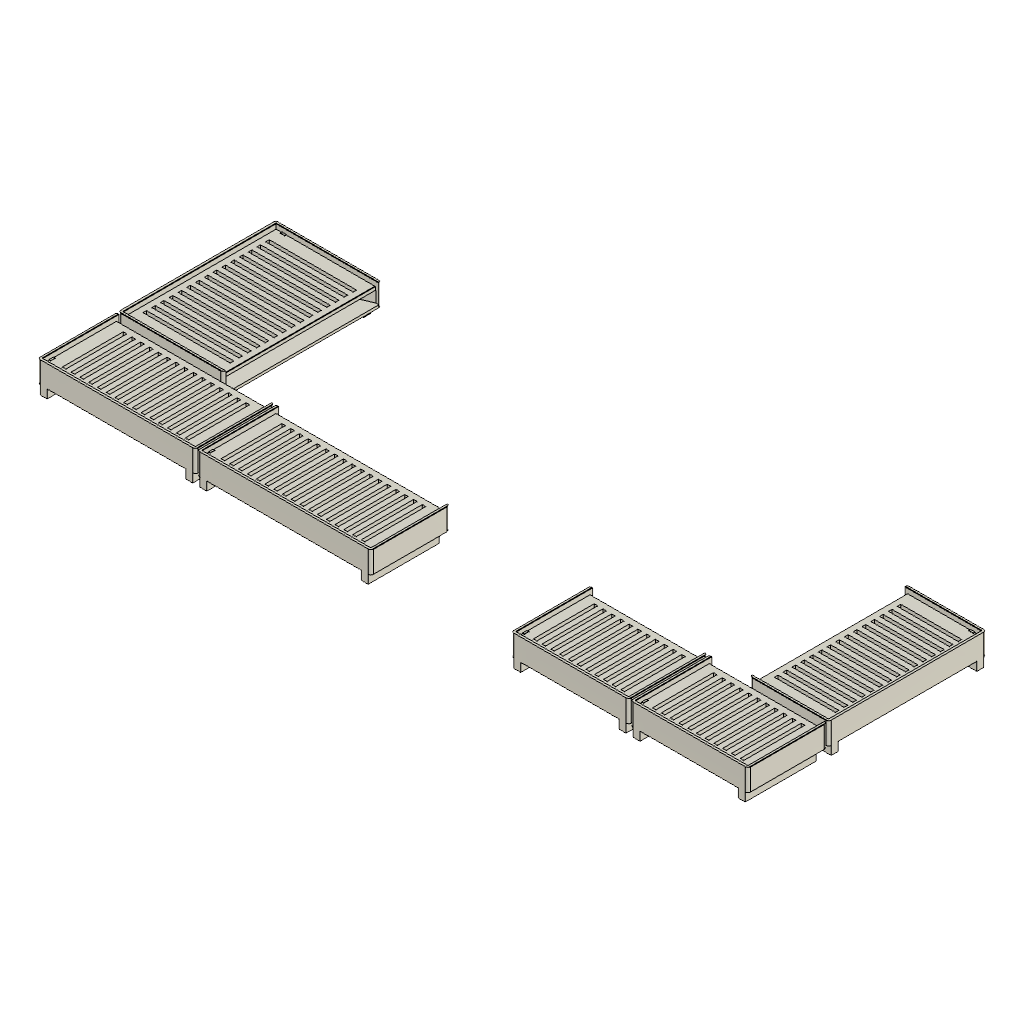
Sink_Organizer_B_R05_Flow_Rim (Autodesk Fusion 360 design; units mm, degrees)
Autodesk Fusion 360 part; units mm, degrees
(part 1 of 5)
ref_plane "工作平面1" through (0, 0, 10) normal (0, 0, 1) x (1, 0, 0) in component "R1_Integrated"
sketch "草图1" plane through (0, 0, 10) normal (0, 0, 1) x (1, 0, 0) in component "R1_Integrated"
  line L0 (590, 50) -> (724, 50)
  line L1 (724, 50) -> (724, 140)
  line L2 (724, 140) -> (590, 140)
  line L3 (590, 140) -> (590, 50)
  dimension "d47" = 590
  dimension "d48" = 50
  dimension "d49" = 134
  dimension "d50" = 90
  constraint horizontal L0
  constraint vertical L1
  constraint horizontal L2
  constraint vertical L3
  measures "d47" horizontal distance of origin L0.start
  measures "d48" vertical distance of origin L0.start
  measures "d49" horizontal distance of L0.start L0.end
  measures "d50" vertical distance of L0.end L1.end
extrude "R05 pan blank" add sketch "草图1" along normal blind 25 makes body 1 in component "R1_Integrated"
fillet "Outside corner rounds" radius 3 4 edges at (590, 140, 22.5) (724, 140, 22.5) (724, 50, 22.5) (590, 50, 22.5) on bodies 1 in component "R1_Integrated"
ref_plane "工作平面2" through (593, 0, 0) normal (1, 0, 0) x (0, 1, 0) in component "R1_Integrated"
sketch "草图2" plane through (593, 0, 0) normal (1, 0, 0) x (0, 0, -1) in component "R1_Integrated"
  line L0 (-22.1441, 53) -> (-13, 140)
  line L1 (-13, 140) -> (-36, 140)
  line L2 (-36, 140) -> (-36, 53)
  line L3 (-36, 53) -> (-22.1441, 53)
  dimension "d59" = 13
  dimension "d61" = 36
  constraint horizontal L1
  constraint vertical L2
  constraint horizontal L3
  measures "d59" horizontal distance of origin L0.end
  measures "d61" horizontal distance of origin L1.end
extrude "R05 continuous slope and open edge" cut sketch "草图2" along normal blind 128 bodies 1 in component "R1_Integrated"
ref_plane "工作平面3" through (0, 0, 10) normal (0, 0, 1) x (1, 0, 0) in component "R1_Integrated"
sketch "草图3" plane through (0, 0, 10) normal (0, 0, 1) x (1, 0, 0) in component "R1_Integrated"
  line L0 (593, 53) -> (600, 65)
  line L1 (600, 65) -> (593, 77)
  line L2 (593, 77) -> (593, 53)
  dimension "d69" = 65
  constraint vertical L2
  measures "d69" vertical distance of origin L0.end
extrude "R05 triangular flow seat 00" add sketch "草图3" along normal blind 16 bodies 1 in component "R1_Integrated"
fillet "R05 soften flow seat tip" radius 1 1 edges at (600, 65, 23.4414) on bodies 1 in component "R1_Integrated"
ref_plane "工作平面4" through (0, 0, 10) normal (0, 0, 1) x (1, 0, 0) in component "R1_Integrated"
sketch "草图4" plane through (0, 0, 10) normal (0, 0, 1) x (1, 0, 0) in component "R1_Integrated"
  line L0 (593, 113) -> (600, 125)
  line L1 (600, 125) -> (593, 137)
  line L2 (593, 137) -> (593, 113)
  dimension "d80" = 125
  constraint vertical L2
  measures "d80" vertical distance of origin L0.end
extrude "R05 triangular flow seat 01" add sketch "草图4" along normal blind 16 bodies 1 in component "R1_Integrated"
fillet "R05 soften flow seat tip (1)" radius 1 1 edges at (600, 125, 20.2883) on bodies 1 in component "R1_Integrated"
ref_plane "工作平面5" through (0, 0, 10) normal (0, 0, 1) x (1, 0, 0) in component "R1_Integrated"
sketch "草图5" plane through (0, 0, 10) normal (0, 0, 1) x (1, 0, 0) in component "R1_Integrated"
  line L0 (721, 53) -> (714, 65)
  line L1 (714, 65) -> (721, 77)
  line L2 (721, 77) -> (721, 53)
  dimension "d88" = 721
  dimension "d90" = 714
  dimension "d91" = 65
  constraint vertical L2
  measures "d88" horizontal distance of origin L0.start
  measures "d90" horizontal distance of origin L0.end
  measures "d91" vertical distance of origin L0.end
extrude "R05 triangular flow seat 10" add sketch "草图5" along normal blind 16 bodies 1 in component "R1_Integrated"
fillet "R05 soften flow seat tip (2)" radius 1 1 edges at (714, 65, 23.4414) on bodies 1 in component "R1_Integrated"
ref_plane "工作平面6" through (0, 0, 10) normal (0, 0, 1) x (1, 0, 0) in component "R1_Integrated"
sketch "草图6" plane through (0, 0, 10) normal (0, 0, 1) x (1, 0, 0) in component "R1_Integrated"
  line L0 (721, 113) -> (714, 125)
  line L1 (714, 125) -> (721, 137)
  line L2 (721, 137) -> (721, 113)
  dimension "d99" = 721
  dimension "d101" = 714
  dimension "d102" = 125
  constraint vertical L2
  measures "d99" horizontal distance of origin L0.start
  measures "d101" horizontal distance of origin L0.end
  measures "d102" vertical distance of origin L0.end
extrude "R05 triangular flow seat 11" add sketch "草图6" along normal blind 16 bodies 1 in component "R1_Integrated"
fillet "R05 soften flow seat tip (3)" radius 1 1 edges at (714, 125, 20.2883) on bodies 1 in component "R1_Integrated"
ref_plane "工作平面7" through (0, 0, 0) normal (0, 0, 1) x (1, 0, 0) in component "R1_Integrated"
sketch "草图7" plane through (0, 0, 0) normal (0, 0, 1) x (1, 0, 0) in component "R1_Integrated"
  line L0 (593, 50) -> (601, 50)
  line L1 (601, 50) -> (601, 131)
  line L2 (601, 131) -> (593, 131)
  line L3 (593, 131) -> (593, 50)
  dimension "d110" = 593
  dimension "d111" = 50
  dimension "d112" = 8
  dimension "d113" = 81
  constraint horizontal L0
  constraint vertical L1
  constraint horizontal L2
  constraint vertical L3
  measures "d110" horizontal distance of origin L0.start
  measures "d111" vertical distance of origin L0.start
  measures "d112" horizontal distance of L0.start L0.end
  measures "d113" vertical distance of L0.end L1.end
extrude "R05 low integral runner 0" add sketch "草图7" along normal blind 10 bodies 1 in component "R1_Integrated"
ref_plane "工作平面8" through (0, 0, 0) normal (0, 0, 1) x (1, 0, 0) in component "R1_Integrated"
sketch "草图8" plane through (0, 0, 0) normal (0, 0, 1) x (1, 0, 0) in component "R1_Integrated"
  line L0 (713, 50) -> (721, 50)
  line L1 (721, 50) -> (721, 131)
  line L2 (721, 131) -> (713, 131)
  line L3 (713, 131) -> (713, 50)
  dimension "d118" = 713
  dimension "d119" = 50
  dimension "d120" = 8
  dimension "d121" = 81
  constraint horizontal L0
  constraint vertical L1
  constraint horizontal L2
  constraint vertical L3
  measures "d118" horizontal distance of origin L0.start
  measures "d119" vertical distance of origin L0.start
  measures "d120" horizontal distance of L0.start L0.end
  measures "d121" vertical distance of L0.end L1.end
extrude "R05 low integral runner 1" add sketch "草图8" along normal blind 10 bodies 1 in component "R1_Integrated"
chamfer "倒角1" distance 0.4 angle 45 5 edges at (593, 96.5, 35) (721, 96.5, 35) (657, 53, 35) (590, 95, 35) (724, 95, 35) on bodies 1 in component "R1_Integrated"
ref_plane "工作平面1" through (0, 0, 26) normal (0, 0, 1) x (1, 0, 0) in component "R1_RemovableGrate"
sketch "草图1 (2)" plane through (0, 0, 26) normal (0, 0, 1) x (1, 0, 0) in component "R1_RemovableGrate"
  line L0 (593.3, 53.3) -> (720.7, 53.3)
  line L1 (720.7, 53.3) -> (720.7, 136.7)
  line L2 (720.7, 136.7) -> (593.3, 136.7)
  line L3 (593.3, 136.7) -> (593.3, 53.3)
  dimension "d129" = 127.4
  dimension "d130" = 83.4
  constraint horizontal L0
  constraint vertical L1
  constraint horizontal L2
  constraint vertical L3
  measures "d129" horizontal distance of L0.start L0.end
  measures "d130" vertical distance of L0.end L1.end
extrude "Horizontal removable deck" add sketch "草图1 (2)" along normal blind 4 separate body makes body 2 in component "R1_RemovableGrate"
ref_plane "工作平面2" through (0, 0, 26) normal (0, 0, 1) x (1, 0, 0) in component "R1_RemovableGrate"
sketch "草图2 (2)" plane through (0, 0, 26) normal (0, 0, 1) x (1, 0, 0) in component "R1_RemovableGrate"
  line L0 (605, 60.3) -> (609, 60.3)
  line L1 (609, 60.3) -> (609, 129.7)
  line L2 (609, 129.7) -> (605, 129.7)
  line L3 (605, 129.7) -> (605, 60.3)
  dimension "d135" = 605
  dimension "d137" = 4
  dimension "d138" = 69.4
  constraint horizontal L0
  constraint vertical L1
  constraint horizontal L2
  constraint vertical L3
  measures "d135" horizontal distance of origin L0.start
  measures "d137" horizontal distance of L0.start L0.end
  measures "d138" vertical distance of L0.end L1.end
extrude "Drain slot 1" cut sketch "草图2 (2)" along normal blind 4 bodies 2 in component "R1_RemovableGrate"
ref_plane "工作平面3" through (0, 0, 26) normal (0, 0, 1) x (1, 0, 0) in component "R1_RemovableGrate"
sketch "草图3 (2)" plane through (0, 0, 26) normal (0, 0, 1) x (1, 0, 0) in component "R1_RemovableGrate"
  line L0 (615, 60.3) -> (619, 60.3)
  line L1 (619, 60.3) -> (619, 129.7)
  line L2 (619, 129.7) -> (615, 129.7)
  line L3 (615, 129.7) -> (615, 60.3)
  dimension "d143" = 615
  dimension "d145" = 4
  dimension "d146" = 69.4
  constraint horizontal L0
  constraint vertical L1
  constraint horizontal L2
  constraint vertical L3
  measures "d143" horizontal distance of origin L0.start
  measures "d145" horizontal distance of L0.start L0.end
  measures "d146" vertical distance of L0.end L1.end
extrude "Drain slot 2" cut sketch "草图3 (2)" along normal blind 4 bodies 2 in component "R1_RemovableGrate"
ref_plane "工作平面4" through (0, 0, 26) normal (0, 0, 1) x (1, 0, 0) in component "R1_RemovableGrate"
sketch "草图4 (2)" plane through (0, 0, 26) normal (0, 0, 1) x (1, 0, 0) in component "R1_RemovableGrate"
  line L0 (625, 60.3) -> (629, 60.3)
  line L1 (629, 60.3) -> (629, 129.7)
  line L2 (629, 129.7) -> (625, 129.7)
  line L3 (625, 129.7) -> (625, 60.3)
  dimension "d151" = 625
  dimension "d153" = 4
  dimension "d154" = 69.4
  constraint horizontal L0
  constraint vertical L1
  constraint horizontal L2
  constraint vertical L3
  measures "d151" horizontal distance of origin L0.start
  measures "d153" horizontal distance of L0.start L0.end
  measures "d154" vertical distance of L0.end L1.end
extrude "Drain slot 3" cut sketch "草图4 (2)" along normal blind 4 bodies 2 in component "R1_RemovableGrate"
ref_plane "工作平面5" through (0, 0, 26) normal (0, 0, 1) x (1, 0, 0) in component "R1_RemovableGrate"
sketch "草图5 (2)" plane through (0, 0, 26) normal (0, 0, 1) x (1, 0, 0) in component "R1_RemovableGrate"
  line L0 (635, 60.3) -> (639, 60.3)
  line L1 (639, 60.3) -> (639, 129.7)
  line L2 (639, 129.7) -> (635, 129.7)
  line L3 (635, 129.7) -> (635, 60.3)
  dimension "d159" = 635
  dimension "d161" = 4
  dimension "d162" = 69.4
  constraint horizontal L0
  constraint vertical L1
  constraint horizontal L2
  constraint vertical L3
  measures "d159" horizontal distance of origin L0.start
  measures "d161" horizontal distance of L0.start L0.end
  measures "d162" vertical distance of L0.end L1.end
extrude "Drain slot 4" cut sketch "草图5 (2)" along normal blind 4 bodies 2 in component "R1_RemovableGrate"
ref_plane "工作平面6" through (0, 0, 26) normal (0, 0, 1) x (1, 0, 0) in component "R1_RemovableGrate"
sketch "草图6 (2)" plane through (0, 0, 26) normal (0, 0, 1) x (1, 0, 0) in component "R1_RemovableGrate"
  line L0 (645, 60.3) -> (649, 60.3)
  line L1 (649, 60.3) -> (649, 129.7)
  line L2 (649, 129.7) -> (645, 129.7)
  line L3 (645, 129.7) -> (645, 60.3)
  dimension "d167" = 645
  dimension "d169" = 4
  dimension "d170" = 69.4
  constraint horizontal L0
  constraint vertical L1
  constraint horizontal L2
  constraint vertical L3
  measures "d167" horizontal distance of origin L0.start
  measures "d169" horizontal distance of L0.start L0.end
  measures "d170" vertical distance of L0.end L1.end
extrude "Drain slot 5" cut sketch "草图6 (2)" along normal blind 4 bodies 2 in component "R1_RemovableGrate"
ref_plane "工作平面7" through (0, 0, 26) normal (0, 0, 1) x (1, 0, 0) in component "R1_RemovableGrate"
sketch "草图7 (2)" plane through (0, 0, 26) normal (0, 0, 1) x (1, 0, 0) in component "R1_RemovableGrate"
  line L0 (655, 60.3) -> (659, 60.3)
  line L1 (659, 60.3) -> (659, 129.7)
  line L2 (659, 129.7) -> (655, 129.7)
  line L3 (655, 129.7) -> (655, 60.3)
  dimension "d175" = 655
  dimension "d177" = 4
  dimension "d178" = 69.4
  constraint horizontal L0
  constraint vertical L1
  constraint horizontal L2
  constraint vertical L3
  measures "d175" horizontal distance of origin L0.start
  measures "d177" horizontal distance of L0.start L0.end
  measures "d178" vertical distance of L0.end L1.end
extrude "Drain slot 6" cut sketch "草图7 (2)" along normal blind 4 bodies 2 in component "R1_RemovableGrate"
ref_plane "工作平面8" through (0, 0, 26) normal (0, 0, 1) x (1, 0, 0) in component "R1_RemovableGrate"
sketch "草图8 (2)" plane through (0, 0, 26) normal (0, 0, 1) x (1, 0, 0) in component "R1_RemovableGrate"
  line L0 (665, 60.3) -> (669, 60.3)
  line L1 (669, 60.3) -> (669, 129.7)
  line L2 (669, 129.7) -> (665, 129.7)
  line L3 (665, 129.7) -> (665, 60.3)
  dimension "d183" = 665
  dimension "d185" = 4
  dimension "d186" = 69.4
  constraint horizontal L0
  constraint vertical L1
  constraint horizontal L2
  constraint vertical L3
  measures "d183" horizontal distance of origin L0.start
  measures "d185" horizontal distance of L0.start L0.end
  measures "d186" vertical distance of L0.end L1.end
extrude "Drain slot 7" cut sketch "草图8 (2)" along normal blind 4 bodies 2 in component "R1_RemovableGrate"
ref_plane "工作平面9" through (0, 0, 26) normal (0, 0, 1) x (1, 0, 0) in component "R1_RemovableGrate"
sketch "草图9" plane through (0, 0, 26) normal (0, 0, 1) x (1, 0, 0) in component "R1_RemovableGrate"
  line L0 (675, 60.3) -> (679, 60.3)
  line L1 (679, 60.3) -> (679, 129.7)
  line L2 (679, 129.7) -> (675, 129.7)
  line L3 (675, 129.7) -> (675, 60.3)
  dimension "d191" = 675
  dimension "d193" = 4
  dimension "d194" = 69.4
  constraint horizontal L0
  constraint vertical L1
  constraint horizontal L2
  constraint vertical L3
  measures "d191" horizontal distance of origin L0.start
  measures "d193" horizontal distance of L0.start L0.end
  measures "d194" vertical distance of L0.end L1.end
extrude "Drain slot 8" cut sketch "草图9" along normal blind 4 bodies 2 in component "R1_RemovableGrate"
ref_plane "工作平面10" through (0, 0, 26) normal (0, 0, 1) x (1, 0, 0) in component "R1_RemovableGrate"
sketch "草图10" plane through (0, 0, 26) normal (0, 0, 1) x (1, 0, 0) in component "R1_RemovableGrate"
  line L0 (685, 60.3) -> (689, 60.3)
  line L1 (689, 60.3) -> (689, 129.7)
  line L2 (689, 129.7) -> (685, 129.7)
  line L3 (685, 129.7) -> (685, 60.3)
  dimension "d199" = 685
  dimension "d201" = 4
  dimension "d202" = 69.4
  constraint horizontal L0
  constraint vertical L1
  constraint horizontal L2
  constraint vertical L3
  measures "d199" horizontal distance of origin L0.start
  measures "d201" horizontal distance of L0.start L0.end
  measures "d202" vertical distance of L0.end L1.end
extrude "Drain slot 9" cut sketch "草图10" along normal blind 4 bodies 2 in component "R1_RemovableGrate"
ref_plane "工作平面11" through (0, 0, 26) normal (0, 0, 1) x (1, 0, 0) in component "R1_RemovableGrate"
sketch "草图11" plane through (0, 0, 26) normal (0, 0, 1) x (1, 0, 0) in component "R1_RemovableGrate"
  line L0 (695, 60.3) -> (699, 60.3)
  line L1 (699, 60.3) -> (699, 129.7)
  line L2 (699, 129.7) -> (695, 129.7)
  line L3 (695, 129.7) -> (695, 60.3)
  dimension "d207" = 695
  dimension "d209" = 4
  dimension "d210" = 69.4
  constraint horizontal L0
  constraint vertical L1
  constraint horizontal L2
  constraint vertical L3
  measures "d207" horizontal distance of origin L0.start
  measures "d209" horizontal distance of L0.start L0.end
  measures "d210" vertical distance of L0.end L1.end
extrude "Drain slot 10" cut sketch "草图11" along normal blind 4 bodies 2 in component "R1_RemovableGrate"
ref_plane "工作平面12" through (0, 0, 26) normal (0, 0, 1) x (1, 0, 0) in component "R1_RemovableGrate"
sketch "草图12" plane through (0, 0, 26) normal (0, 0, 1) x (1, 0, 0) in component "R1_RemovableGrate"
  line L0 (705, 60.3) -> (709, 60.3)
  line L1 (709, 60.3) -> (709, 129.7)
  line L2 (709, 129.7) -> (705, 129.7)
  line L3 (705, 129.7) -> (705, 60.3)
  dimension "d215" = 705
  dimension "d217" = 4
  dimension "d218" = 69.4
  constraint horizontal L0
  constraint vertical L1
  constraint horizontal L2
  constraint vertical L3
  measures "d215" horizontal distance of origin L0.start
  measures "d217" horizontal distance of L0.start L0.end
  measures "d218" vertical distance of L0.end L1.end
extrude "Drain slot 11" cut sketch "草图12" along normal blind 4 bodies 2 in component "R1_RemovableGrate"
chamfer "倒角1'" distance 0.4 angle 45 4 edges at (657, 136.7, 30) (720.7, 95, 30) (657, 53.3, 30) (593.3, 95, 30) on bodies 2 in component "R1_RemovableGrate"
ref_plane "工作平面1" through (0, 0, 10) normal (0, 0, 1) x (1, 0, 0) in component "L1_Integrated"
sketch "草图1 (3)" plane through (0, 0, 10) normal (0, 0, 1) x (1, 0, 0) in component "L1_Integrated"
  line L0 (50, 50) -> (230, 50)
  line L1 (230, 50) -> (230, 140)
  line L2 (230, 140) -> (50, 140)
  line L3 (50, 140) -> (50, 50)
  dimension "d224" = 50
  dimension "d225" = 50
  dimension "d226" = 180
  dimension "d227" = 90
  constraint horizontal L0
  constraint vertical L1
  constraint horizontal L2
  constraint vertical L3
  measures "d224" horizontal distance of origin L0.start
  measures "d225" vertical distance of origin L0.start
  measures "d226" horizontal distance of L0.start L0.end
  measures "d227" vertical distance of L0.end L1.end
extrude "R05 pan blank'" add sketch "草图1 (3)" along normal blind 25 separate body makes body 3 in component "L1_Integrated"
fillet "Outside corner rounds'" radius 3 4 edges at (50, 140, 22.5) (230, 140, 22.5) (230, 50, 22.5) (50, 50, 22.5) on bodies 3 in component "L1_Integrated"
ref_plane "工作平面2" through (53, 0, 0) normal (1, 0, 0) x (0, 1, 0) in component "L1_Integrated"
sketch "草图2 (3)" plane through (53, 0, 0) normal (1, 0, 0) x (0, 0, -1) in component "L1_Integrated"
  line L0 (-22.1441, 53) -> (-13, 140)
  line L1 (-13, 140) -> (-36, 140)
  line L2 (-36, 140) -> (-36, 53)
  line L3 (-36, 53) -> (-22.1441, 53)
  dimension "d236" = 13
  dimension "d238" = 36
  constraint horizontal L1
  constraint vertical L2
  constraint horizontal L3
  measures "d236" horizontal distance of origin L0.end
  measures "d238" horizontal distance of origin L1.end
extrude "R05 continuous slope and open edge'" cut sketch "草图2 (3)" along normal blind 174 bodies 3 in component "L1_Integrated"
ref_plane "工作平面3" through (0, 0, 10) normal (0, 0, 1) x (1, 0, 0) in component "L1_Integrated"
sketch "草图3 (3)" plane through (0, 0, 10) normal (0, 0, 1) x (1, 0, 0) in component "L1_Integrated"
  line L0 (53, 53) -> (60, 65)
  line L1 (60, 65) -> (53, 77)
  line L2 (53, 77) -> (53, 53)
  dimension "d246" = 65
  constraint vertical L2
  measures "d246" vertical distance of origin L0.end
extrude "R05 triangular flow seat 00'" add sketch "草图3 (3)" along normal blind 16 bodies 3 in component "L1_Integrated"
fillet "R05 soften flow seat tip'" radius 1 1 edges at (60, 65, 23.4414) on bodies 3 in component "L1_Integrated"
ref_plane "工作平面4" through (0, 0, 10) normal (0, 0, 1) x (1, 0, 0) in component "L1_Integrated"
sketch "草图4 (3)" plane through (0, 0, 10) normal (0, 0, 1) x (1, 0, 0) in component "L1_Integrated"
  line L0 (53, 113) -> (60, 125)
  line L1 (60, 125) -> (53, 137)
  line L2 (53, 137) -> (53, 113)
  dimension "d257" = 125
  constraint vertical L2
  measures "d257" vertical distance of origin L0.end
extrude "R05 triangular flow seat 01'" add sketch "草图4 (3)" along normal blind 16 bodies 3 in component "L1_Integrated"
fillet "R05 soften flow seat tip (1)'" radius 1 1 edges at (60, 125, 20.2883) on bodies 3 in component "L1_Integrated"
ref_plane "工作平面5" through (0, 0, 10) normal (0, 0, 1) x (1, 0, 0) in component "L1_Integrated"
sketch "草图5 (3)" plane through (0, 0, 10) normal (0, 0, 1) x (1, 0, 0) in component "L1_Integrated"
  line L0 (227, 53) -> (220, 65)
  line L1 (220, 65) -> (227, 77)
  line L2 (227, 77) -> (227, 53)
  dimension "d268" = 65
  constraint vertical L2
  measures "d268" vertical distance of origin L0.end
extrude "R05 triangular flow seat 10'" add sketch "草图5 (3)" along normal blind 16 bodies 3 in component "L1_Integrated"
fillet "R05 soften flow seat tip (2)'" radius 1 1 edges at (220, 65, 23.4414) on bodies 3 in component "L1_Integrated"
ref_plane "工作平面6" through (0, 0, 10) normal (0, 0, 1) x (1, 0, 0) in component "L1_Integrated"
sketch "草图6 (3)" plane through (0, 0, 10) normal (0, 0, 1) x (1, 0, 0) in component "L1_Integrated"
  line L0 (227, 113) -> (220, 125)
  line L1 (220, 125) -> (227, 137)
  line L2 (227, 137) -> (227, 113)
  dimension "d279" = 125
  constraint vertical L2
  measures "d279" vertical distance of origin L0.end
extrude "R05 triangular flow seat 11'" add sketch "草图6 (3)" along normal blind 16 bodies 3 in component "L1_Integrated"
fillet "R05 soften flow seat tip (3)'" radius 1 1 edges at (220, 125, 20.2883) on bodies 3 in component "L1_Integrated"
ref_plane "工作平面7" through (0, 0, 0) normal (0, 0, 1) x (1, 0, 0) in component "L1_Integrated"
sketch "草图7 (3)" plane through (0, 0, 0) normal (0, 0, 1) x (1, 0, 0) in component "L1_Integrated"
  line L0 (53, 50) -> (61, 50)
  line L1 (61, 50) -> (61, 131)
  line L2 (61, 131) -> (53, 131)
  line L3 (53, 131) -> (53, 50)
  dimension "d287" = 53
  dimension "d288" = 50
  dimension "d289" = 8
  dimension "d290" = 81
  constraint horizontal L0
  constraint vertical L1
  constraint horizontal L2
  constraint vertical L3
  measures "d287" horizontal distance of origin L0.start
  measures "d288" vertical distance of origin L0.start
  measures "d289" horizontal distance of L0.start L0.end
  measures "d290" vertical distance of L0.end L1.end
extrude "R05 low integral runner 0'" add sketch "草图7 (3)" along normal blind 10 bodies 3 in component "L1_Integrated"
ref_plane "工作平面8" through (0, 0, 0) normal (0, 0, 1) x (1, 0, 0) in component "L1_Integrated"
sketch "草图8 (3)" plane through (0, 0, 0) normal (0, 0, 1) x (1, 0, 0) in component "L1_Integrated"
  line L0 (219, 50) -> (227, 50)
  line L1 (227, 50) -> (227, 131)
  line L2 (227, 131) -> (219, 131)
  line L3 (219, 131) -> (219, 50)
  dimension "d295" = 219
  dimension "d296" = 50
  dimension "d297" = 8
  dimension "d298" = 81
  constraint horizontal L0
  constraint vertical L1
  constraint horizontal L2
  constraint vertical L3
  measures "d295" horizontal distance of origin L0.start
  measures "d296" vertical distance of origin L0.start
  measures "d297" horizontal distance of L0.start L0.end
  measures "d298" vertical distance of L0.end L1.end
extrude "R05 low integral runner 1'" add sketch "草图8 (3)" along normal blind 10 bodies 3 in component "L1_Integrated"
chamfer "倒角1''" distance 0.4 angle 45 5 edges at (53, 96.5, 35) (227, 96.5, 35) (140, 53, 35) (50, 95, 35) (230, 95, 35) on bodies 3 in component "L1_Integrated"
ref_plane "工作平面1" through (0, 0, 26) normal (0, 0, 1) x (1, 0, 0) in component "L1_RemovableGrate"
sketch "草图1 (4)" plane through (0, 0, 26) normal (0, 0, 1) x (1, 0, 0) in component "L1_RemovableGrate"
  line L0 (53.3, 53.3) -> (226.7, 53.3)
  line L1 (226.7, 53.3) -> (226.7, 136.7)
  line L2 (226.7, 136.7) -> (53.3, 136.7)
  line L3 (53.3, 136.7) -> (53.3, 53.3)
  dimension "d306" = 173.4
  dimension "d307" = 83.4
  constraint horizontal L0
  constraint vertical L1
  constraint horizontal L2
  constraint vertical L3
  measures "d306" horizontal distance of L0.start L0.end
  measures "d307" vertical distance of L0.end L1.end
extrude "Horizontal removable deck'" add sketch "草图1 (4)" along normal blind 4 separate body makes body 4 in component "L1_RemovableGrate"
ref_plane "工作平面2" through (0, 0, 26) normal (0, 0, 1) x (1, 0, 0) in component "L1_RemovableGrate"
sketch "草图2 (4)" plane through (0, 0, 26) normal (0, 0, 1) x (1, 0, 0) in component "L1_RemovableGrate"
  line L0 (68, 60.3) -> (72, 60.3)
  line L1 (72, 60.3) -> (72, 129.7)
  line L2 (72, 129.7) -> (68, 129.7)
  line L3 (68, 129.7) -> (68, 60.3)
  dimension "d312" = 68
  dimension "d314" = 4
  dimension "d315" = 69.4
  constraint horizontal L0
  constraint vertical L1
  constraint horizontal L2
  constraint vertical L3
  measures "d312" horizontal distance of origin L0.start
  measures "d314" horizontal distance of L0.start L0.end
  measures "d315" vertical distance of L0.end L1.end
extrude "Drain slot 1'" cut sketch "草图2 (4)" along normal blind 4 bodies 4 in component "L1_RemovableGrate"
ref_plane "工作平面3" through (0, 0, 26) normal (0, 0, 1) x (1, 0, 0) in component "L1_RemovableGrate"
sketch "草图3 (4)" plane through (0, 0, 26) normal (0, 0, 1) x (1, 0, 0) in component "L1_RemovableGrate"
  line L0 (78, 60.3) -> (82, 60.3)
  line L1 (82, 60.3) -> (82, 129.7)
  line L2 (82, 129.7) -> (78, 129.7)
  line L3 (78, 129.7) -> (78, 60.3)
  dimension "d320" = 78
  dimension "d322" = 4
  dimension "d323" = 69.4
  constraint horizontal L0
  constraint vertical L1
  constraint horizontal L2
  constraint vertical L3
  measures "d320" horizontal distance of origin L0.start
  measures "d322" horizontal distance of L0.start L0.end
  measures "d323" vertical distance of L0.end L1.end
extrude "Drain slot 2'" cut sketch "草图3 (4)" along normal blind 4 bodies 4 in component "L1_RemovableGrate"
ref_plane "工作平面4" through (0, 0, 26) normal (0, 0, 1) x (1, 0, 0) in component "L1_RemovableGrate"
sketch "草图4 (4)" plane through (0, 0, 26) normal (0, 0, 1) x (1, 0, 0) in component "L1_RemovableGrate"
  line L0 (88, 60.3) -> (92, 60.3)
  line L1 (92, 60.3) -> (92, 129.7)
  line L2 (92, 129.7) -> (88, 129.7)
  line L3 (88, 129.7) -> (88, 60.3)
  dimension "d328" = 88
  dimension "d330" = 4
  dimension "d331" = 69.4
  constraint horizontal L0
  constraint vertical L1
  constraint horizontal L2
  constraint vertical L3
  measures "d328" horizontal distance of origin L0.start
  measures "d330" horizontal distance of L0.start L0.end
  measures "d331" vertical distance of L0.end L1.end
extrude "Drain slot 3'" cut sketch "草图4 (4)" along normal blind 4 bodies 4 in component "L1_RemovableGrate"
ref_plane "工作平面5" through (0, 0, 26) normal (0, 0, 1) x (1, 0, 0) in component "L1_RemovableGrate"
sketch "草图5 (4)" plane through (0, 0, 26) normal (0, 0, 1) x (1, 0, 0) in component "L1_RemovableGrate"
  line L0 (98, 60.3) -> (102, 60.3)
  line L1 (102, 60.3) -> (102, 129.7)
  line L2 (102, 129.7) -> (98, 129.7)
  line L3 (98, 129.7) -> (98, 60.3)
  dimension "d336" = 98
  dimension "d338" = 4
  dimension "d339" = 69.4
  constraint horizontal L0
  constraint vertical L1
  constraint horizontal L2
  constraint vertical L3
  measures "d336" horizontal distance of origin L0.start
  measures "d338" horizontal distance of L0.start L0.end
  measures "d339" vertical distance of L0.end L1.end
extrude "Drain slot 4'" cut sketch "草图5 (4)" along normal blind 4 bodies 4 in component "L1_RemovableGrate"
ref_plane "工作平面6" through (0, 0, 26) normal (0, 0, 1) x (1, 0, 0) in component "L1_RemovableGrate"
sketch "草图6 (4)" plane through (0, 0, 26) normal (0, 0, 1) x (1, 0, 0) in component "L1_RemovableGrate"
  line L0 (108, 60.3) -> (112, 60.3)
  line L1 (112, 60.3) -> (112, 129.7)
  line L2 (112, 129.7) -> (108, 129.7)
  line L3 (108, 129.7) -> (108, 60.3)
  dimension "d344" = 108
  dimension "d346" = 4
  dimension "d347" = 69.4
  constraint horizontal L0
  constraint vertical L1
  constraint horizontal L2
  constraint vertical L3
  measures "d344" horizontal distance of origin L0.start
  measures "d346" horizontal distance of L0.start L0.end
  measures "d347" vertical distance of L0.end L1.end
extrude "Drain slot 5'" cut sketch "草图6 (4)" along normal blind 4 bodies 4 in component "L1_RemovableGrate"
ref_plane "工作平面7" through (0, 0, 26) normal (0, 0, 1) x (1, 0, 0) in component "L1_RemovableGrate"
sketch "草图7 (4)" plane through (0, 0, 26) normal (0, 0, 1) x (1, 0, 0) in component "L1_RemovableGrate"
  line L0 (118, 60.3) -> (122, 60.3)
  line L1 (122, 60.3) -> (122, 129.7)
  line L2 (122, 129.7) -> (118, 129.7)
  line L3 (118, 129.7) -> (118, 60.3)
  dimension "d352" = 118
  dimension "d354" = 4
  dimension "d355" = 69.4
  constraint horizontal L0
  constraint vertical L1
  constraint horizontal L2
  constraint vertical L3
  measures "d352" horizontal distance of origin L0.start
  measures "d354" horizontal distance of L0.start L0.end
  measures "d355" vertical distance of L0.end L1.end
extrude "Drain slot 6'" cut sketch "草图7 (4)" along normal blind 4 bodies 4 in component "L1_RemovableGrate"
ref_plane "工作平面8" through (0, 0, 26) normal (0, 0, 1) x (1, 0, 0) in component "L1_RemovableGrate"
sketch "草图8 (4)" plane through (0, 0, 26) normal (0, 0, 1) x (1, 0, 0) in component "L1_RemovableGrate"
  line L0 (128, 60.3) -> (132, 60.3)
  line L1 (132, 60.3) -> (132, 129.7)
  line L2 (132, 129.7) -> (128, 129.7)
  line L3 (128, 129.7) -> (128, 60.3)
  dimension "d360" = 128
  dimension "d362" = 4
  dimension "d363" = 69.4
  constraint horizontal L0
  constraint vertical L1
  constraint horizontal L2
  constraint vertical L3
  measures "d360" horizontal distance of origin L0.start
  measures "d362" horizontal distance of L0.start L0.end
  measures "d363" vertical distance of L0.end L1.end
extrude "Drain slot 7'" cut sketch "草图8 (4)" along normal blind 4 bodies 4 in component "L1_RemovableGrate"
ref_plane "工作平面9" through (0, 0, 26) normal (0, 0, 1) x (1, 0, 0) in component "L1_RemovableGrate"
sketch "草图9 (2)" plane through (0, 0, 26) normal (0, 0, 1) x (1, 0, 0) in component "L1_RemovableGrate"
  line L0 (138, 60.3) -> (142, 60.3)
  line L1 (142, 60.3) -> (142, 129.7)
  line L2 (142, 129.7) -> (138, 129.7)
  line L3 (138, 129.7) -> (138, 60.3)
  dimension "d368" = 138
  dimension "d370" = 4
  dimension "d371" = 69.4
  constraint horizontal L0
  constraint vertical L1
  constraint horizontal L2
  constraint vertical L3
  measures "d368" horizontal distance of origin L0.start
  measures "d370" horizontal distance of L0.start L0.end
  measures "d371" vertical distance of L0.end L1.end
extrude "Drain slot 8'" cut sketch "草图9 (2)" along normal blind 4 bodies 4 in component "L1_RemovableGrate"
ref_plane "工作平面10" through (0, 0, 26) normal (0, 0, 1) x (1, 0, 0) in component "L1_RemovableGrate"
sketch "草图10 (2)" plane through (0, 0, 26) normal (0, 0, 1) x (1, 0, 0) in component "L1_RemovableGrate"
  line L0 (148, 60.3) -> (152, 60.3)
  line L1 (152, 60.3) -> (152, 129.7)
  line L2 (152, 129.7) -> (148, 129.7)
  line L3 (148, 129.7) -> (148, 60.3)
  dimension "d376" = 148
  dimension "d378" = 4
  dimension "d379" = 69.4
  constraint horizontal L0
  constraint vertical L1
  constraint horizontal L2
  constraint vertical L3
  measures "d376" horizontal distance of origin L0.start
  measures "d378" horizontal distance of L0.start L0.end
  measures "d379" vertical distance of L0.end L1.end
extrude "Drain slot 9'" cut sketch "草图10 (2)" along normal blind 4 bodies 4 in component "L1_RemovableGrate"
ref_plane "工作平面11" through (0, 0, 26) normal (0, 0, 1) x (1, 0, 0) in component "L1_RemovableGrate"
sketch "草图11 (2)" plane through (0, 0, 26) normal (0, 0, 1) x (1, 0, 0) in component "L1_RemovableGrate"
  line L0 (158, 60.3) -> (162, 60.3)
  line L1 (162, 60.3) -> (162, 129.7)
  line L2 (162, 129.7) -> (158, 129.7)
  line L3 (158, 129.7) -> (158, 60.3)
  dimension "d384" = 158
  dimension "d386" = 4
  dimension "d387" = 69.4
  constraint horizontal L0
  constraint vertical L1
  constraint horizontal L2
  constraint vertical L3
  measures "d384" horizontal distance of origin L0.start
  measures "d386" horizontal distance of L0.start L0.end
  measures "d387" vertical distance of L0.end L1.end
extrude "Drain slot 10'" cut sketch "草图11 (2)" along normal blind 4 bodies 4 in component "L1_RemovableGrate"
ref_plane "工作平面12" through (0, 0, 26) normal (0, 0, 1) x (1, 0, 0) in component "L1_RemovableGrate"
sketch "草图12 (2)" plane through (0, 0, 26) normal (0, 0, 1) x (1, 0, 0) in component "L1_RemovableGrate"
  line L0 (168, 60.3) -> (172, 60.3)
  line L1 (172, 60.3) -> (172, 129.7)
  line L2 (172, 129.7) -> (168, 129.7)
  line L3 (168, 129.7) -> (168, 60.3)
  dimension "d392" = 168
  dimension "d394" = 4
  dimension "d395" = 69.4
  constraint horizontal L0
  constraint vertical L1
  constraint horizontal L2
  constraint vertical L3
  measures "d392" horizontal distance of origin L0.start
  measures "d394" horizontal distance of L0.start L0.end
  measures "d395" vertical distance of L0.end L1.end
extrude "Drain slot 11'" cut sketch "草图12 (2)" along normal blind 4 bodies 4 in component "L1_RemovableGrate"
ref_plane "工作平面13" through (0, 0, 26) normal (0, 0, 1) x (1, 0, 0) in component "L1_RemovableGrate"
sketch "草图13" plane through (0, 0, 26) normal (0, 0, 1) x (1, 0, 0) in component "L1_RemovableGrate"
  line L0 (178, 60.3) -> (182, 60.3)
  line L1 (182, 60.3) -> (182, 129.7)
  line L2 (182, 129.7) -> (178, 129.7)
  line L3 (178, 129.7) -> (178, 60.3)
  dimension "d400" = 178
  dimension "d402" = 4
  dimension "d403" = 69.4
  constraint horizontal L0
  constraint vertical L1
  constraint horizontal L2
  constraint vertical L3
  measures "d400" horizontal distance of origin L0.start
  measures "d402" horizontal distance of L0.start L0.end
  measures "d403" vertical distance of L0.end L1.end
extrude "Drain slot 12" cut sketch "草图13" along normal blind 4 bodies 4 in component "L1_RemovableGrate"
ref_plane "工作平面14" through (0, 0, 26) normal (0, 0, 1) x (1, 0, 0) in component "L1_RemovableGrate"
sketch "草图14" plane through (0, 0, 26) normal (0, 0, 1) x (1, 0, 0) in component "L1_RemovableGrate"
  line L0 (188, 60.3) -> (192, 60.3)
  line L1 (192, 60.3) -> (192, 129.7)
  line L2 (192, 129.7) -> (188, 129.7)
  line L3 (188, 129.7) -> (188, 60.3)
  dimension "d408" = 188
  dimension "d410" = 4
  dimension "d411" = 69.4
  constraint horizontal L0
  constraint vertical L1
  constraint horizontal L2
  constraint vertical L3
  measures "d408" horizontal distance of origin L0.start
  measures "d410" horizontal distance of L0.start L0.end
  measures "d411" vertical distance of L0.end L1.end
extrude "Drain slot 13" cut sketch "草图14" along normal blind 4 bodies 4 in component "L1_RemovableGrate"
ref_plane "工作平面15" through (0, 0, 26) normal (0, 0, 1) x (1, 0, 0) in component "L1_RemovableGrate"
sketch "草图15" plane through (0, 0, 26) normal (0, 0, 1) x (1, 0, 0) in component "L1_RemovableGrate"
  line L0 (198, 60.3) -> (202, 60.3)
  line L1 (202, 60.3) -> (202, 129.7)
  line L2 (202, 129.7) -> (198, 129.7)
  line L3 (198, 129.7) -> (198, 60.3)
  dimension "d416" = 198
  dimension "d418" = 4
  dimension "d419" = 69.4
  constraint horizontal L0
  constraint vertical L1
  constraint horizontal L2
  constraint vertical L3
  measures "d416" horizontal distance of origin L0.start
  measures "d418" horizontal distance of L0.start L0.end
  measures "d419" vertical distance of L0.end L1.end
extrude "Drain slot 14" cut sketch "草图15" along normal blind 4 bodies 4 in component "L1_RemovableGrate"
ref_plane "工作平面16" through (0, 0, 26) normal (0, 0, 1) x (1, 0, 0) in component "L1_RemovableGrate"
sketch "草图16" plane through (0, 0, 26) normal (0, 0, 1) x (1, 0, 0) in component "L1_RemovableGrate"
  line L0 (208, 60.3) -> (212, 60.3)
  line L1 (212, 60.3) -> (212, 129.7)
  line L2 (212, 129.7) -> (208, 129.7)
  line L3 (208, 129.7) -> (208, 60.3)
  dimension "d424" = 208
  dimension "d426" = 4
  dimension "d427" = 69.4
  constraint horizontal L0
  constraint vertical L1
  constraint horizontal L2
  constraint vertical L3
  measures "d424" horizontal distance of origin L0.start
  measures "d426" horizontal distance of L0.start L0.end
  measures "d427" vertical distance of L0.end L1.end
extrude "Drain slot 15" cut sketch "草图16" along normal blind 4 bodies 4 in component "L1_RemovableGrate"
chamfer "倒角1'''" distance 0.4 angle 45 4 edges at (140, 136.7, 30) (226.7, 95, 30) (140, 53.3, 30) (53.3, 95, 30) on bodies 4 in component "L1_RemovableGrate"
ref_plane "工作平面1" through (0, 0, 10) normal (0, 0, 1) x (1, 0, 0) in component "L2_Integrated"
sketch "草图1 (5)" plane through (0, 0, 10) normal (0, 0, 1) x (1, 0, 0) in component "L2_Integrated"
  line L0 (232, 50) -> (430, 50)
  line L1 (430, 50) -> (430, 140)
  line L2 (430, 140) -> (232, 140)
  line L3 (232, 140) -> (232, 50)
  dimension "d433" = 232
  dimension "d434" = 50
  dimension "d435" = 198
  dimension "d436" = 90
  constraint horizontal L0
  constraint vertical L1
  constraint horizontal L2
  constraint vertical L3
  measures "d433" horizontal distance of origin L0.start
  measures "d434" vertical distance of origin L0.start
  measures "d435" horizontal distance of L0.start L0.end
  measures "d436" vertical distance of L0.end L1.end
extrude "R05 pan blank''" add sketch "草图1 (5)" along normal blind 25 separate body makes body 5 in component "L2_Integrated"
fillet "Outside corner rounds''" radius 3 4 edges at (232, 140, 22.5) (430, 140, 22.5) (430, 50, 22.5) (232, 50, 22.5) on bodies 5 in component "L2_Integrated"
ref_plane "工作平面2" through (235, 0, 0) normal (1, 0, 0) x (0, 1, 0) in component "L2_Integrated"
sketch "草图2 (5)" plane through (235, 0, 0) normal (1, 0, 0) x (0, 0, -1) in component "L2_Integrated"
  line L0 (-22.1441, 53) -> (-13, 140)
  line L1 (-13, 140) -> (-36, 140)
  line L2 (-36, 140) -> (-36, 53)
  line L3 (-36, 53) -> (-22.1441, 53)
  dimension "d445" = 13
  dimension "d447" = 36
  constraint horizontal L1
  constraint vertical L2
  constraint horizontal L3
  measures "d445" horizontal distance of origin L0.end
  measures "d447" horizontal distance of origin L1.end
extrude "R05 continuous slope and open edge''" cut sketch "草图2 (5)" along normal blind 192 bodies 5 in component "L2_Integrated"
ref_plane "工作平面3" through (0, 0, 10) normal (0, 0, 1) x (1, 0, 0) in component "L2_Integrated"
sketch "草图3 (5)" plane through (0, 0, 10) normal (0, 0, 1) x (1, 0, 0) in component "L2_Integrated"
  line L0 (235, 53) -> (242, 65)
  line L1 (242, 65) -> (235, 77)
  line L2 (235, 77) -> (235, 53)
  dimension "d455" = 65
  constraint vertical L2
  measures "d455" vertical distance of origin L0.end
extrude "R05 triangular flow seat 00''" add sketch "草图3 (5)" along normal blind 16 bodies 5 in component "L2_Integrated"
fillet "R05 soften flow seat tip''" radius 1 1 edges at (242, 65, 23.4414) on bodies 5 in component "L2_Integrated"
ref_plane "工作平面4" through (0, 0, 10) normal (0, 0, 1) x (1, 0, 0) in component "L2_Integrated"
sketch "草图4 (5)" plane through (0, 0, 10) normal (0, 0, 1) x (1, 0, 0) in component "L2_Integrated"
  line L0 (235, 113) -> (242, 125)
  line L1 (242, 125) -> (235, 137)
  line L2 (235, 137) -> (235, 113)
  dimension "d466" = 125
  constraint vertical L2
  measures "d466" vertical distance of origin L0.end
extrude "R05 triangular flow seat 01''" add sketch "草图4 (5)" along normal blind 16 bodies 5 in component "L2_Integrated"
fillet "R05 soften flow seat tip (1)''" radius 1 1 edges at (242, 125, 20.2883) on bodies 5 in component "L2_Integrated"
ref_plane "工作平面5" through (0, 0, 10) normal (0, 0, 1) x (1, 0, 0) in component "L2_Integrated"
sketch "草图5 (5)" plane through (0, 0, 10) normal (0, 0, 1) x (1, 0, 0) in component "L2_Integrated"
  line L0 (427, 53) -> (420, 65)
  line L1 (420, 65) -> (427, 77)
  line L2 (427, 77) -> (427, 53)
  dimension "d474" = 427
  dimension "d476" = 420
  dimension "d477" = 65
  constraint vertical L2
  measures "d474" horizontal distance of origin L0.start
  measures "d476" horizontal distance of origin L0.end
  measures "d477" vertical distance of origin L0.end
extrude "R05 triangular flow seat 10''" add sketch "草图5 (5)" along normal blind 16 bodies 5 in component "L2_Integrated"
fillet "R05 soften flow seat tip (2)''" radius 1 1 edges at (420, 65, 23.4414) on bodies 5 in component "L2_Integrated"
ref_plane "工作平面6" through (0, 0, 10) normal (0, 0, 1) x (1, 0, 0) in component "L2_Integrated"
sketch "草图6 (5)" plane through (0, 0, 10) normal (0, 0, 1) x (1, 0, 0) in component "L2_Integrated"
  line L0 (427, 113) -> (420, 125)
  line L1 (420, 125) -> (427, 137)
  line L2 (427, 137) -> (427, 113)
  dimension "d485" = 427
  dimension "d487" = 420
  dimension "d488" = 125
  constraint vertical L2
  measures "d485" horizontal distance of origin L0.start
  measures "d487" horizontal distance of origin L0.end
  measures "d488" vertical distance of origin L0.end
extrude "R05 triangular flow seat 11''" add sketch "草图6 (5)" along normal blind 16 bodies 5 in component "L2_Integrated"
fillet "R05 soften flow seat tip (3)''" radius 1 1 edges at (420, 125, 20.2883) on bodies 5 in component "L2_Integrated"
ref_plane "工作平面7" through (0, 0, 0) normal (0, 0, 1) x (1, 0, 0) in component "L2_Integrated"
sketch "草图7 (5)" plane through (0, 0, 0) normal (0, 0, 1) x (1, 0, 0) in component "L2_Integrated"
  line L0 (235, 50) -> (243, 50)
  line L1 (243, 50) -> (243, 131)
  line L2 (243, 131) -> (235, 131)
  line L3 (235, 131) -> (235, 50)
  dimension "d496" = 235
  dimension "d497" = 50
  dimension "d498" = 8
  dimension "d499" = 81
  constraint horizontal L0
  constraint vertical L1
  constraint horizontal L2
  constraint vertical L3
  measures "d496" horizontal distance of origin L0.start
  measures "d497" vertical distance of origin L0.start
  measures "d498" horizontal distance of L0.start L0.end
  measures "d499" vertical distance of L0.end L1.end
extrude "R05 low integral runner 0''" add sketch "草图7 (5)" along normal blind 10 bodies 5 in component "L2_Integrated"
ref_plane "工作平面8" through (0, 0, 0) normal (0, 0, 1) x (1, 0, 0) in component "L2_Integrated"
sketch "草图8 (5)" plane through (0, 0, 0) normal (0, 0, 1) x (1, 0, 0) in component "L2_Integrated"
  line L0 (419, 50) -> (427, 50)
  line L1 (427, 50) -> (427, 131)
  line L2 (427, 131) -> (419, 131)
  line L3 (419, 131) -> (419, 50)
  dimension "d504" = 419
  dimension "d505" = 50
  dimension "d506" = 8
  dimension "d507" = 81
  constraint horizontal L0
  constraint vertical L1
  constraint horizontal L2
  constraint vertical L3
  measures "d504" horizontal distance of origin L0.start
  measures "d505" vertical distance of origin L0.start
  measures "d506" horizontal distance of L0.start L0.end
  measures "d507" vertical distance of L0.end L1.end
extrude "R05 low integral runner 1''" add sketch "草图8 (5)" along normal blind 10 bodies 5 in component "L2_Integrated"
chamfer "倒角1''''" distance 0.4 angle 45 5 edges at (235, 96.5, 35) (427, 96.5, 35) (331, 53, 35) (232, 95, 35) (430, 95, 35) on bodies 5 in component "L2_Integrated"
ref_plane "工作平面1" through (0, 0, 26) normal (0, 0, 1) x (1, 0, 0) in component "L2_RemovableGrate"
sketch "草图1 (6)" plane through (0, 0, 26) normal (0, 0, 1) x (1, 0, 0) in component "L2_RemovableGrate"
  line L0 (235.3, 53.3) -> (426.7, 53.3)
  line L1 (426.7, 53.3) -> (426.7, 136.7)
  line L2 (426.7, 136.7) -> (235.3, 136.7)
  line L3 (235.3, 136.7) -> (235.3, 53.3)
  dimension "d515" = 191.4
  dimension "d516" = 83.4
  constraint horizontal L0
  constraint vertical L1
  constraint horizontal L2
  constraint vertical L3
  measures "d515" horizontal distance of L0.start L0.end
  measures "d516" vertical distance of L0.end L1.end
extrude "Horizontal removable deck''" add sketch "草图1 (6)" along normal blind 4 separate body makes body 6 in component "L2_RemovableGrate"
ref_plane "工作平面2" through (0, 0, 26) normal (0, 0, 1) x (1, 0, 0) in component "L2_RemovableGrate"
sketch "草图2 (6)" plane through (0, 0, 26) normal (0, 0, 1) x (1, 0, 0) in component "L2_RemovableGrate"
  line L0 (249, 60.3) -> (253, 60.3)
  line L1 (253, 60.3) -> (253, 129.7)
  line L2 (253, 129.7) -> (249, 129.7)
  line L3 (249, 129.7) -> (249, 60.3)
  dimension "d521" = 249
  dimension "d523" = 4
  dimension "d524" = 69.4
  constraint horizontal L0
  constraint vertical L1
  constraint horizontal L2
  constraint vertical L3
  measures "d521" horizontal distance of origin L0.start
  measures "d523" horizontal distance of L0.start L0.end
  measures "d524" vertical distance of L0.end L1.end
extrude "Drain slot 1''" cut sketch "草图2 (6)" along normal blind 4 bodies 6 in component "L2_RemovableGrate"
ref_plane "工作平面3" through (0, 0, 26) normal (0, 0, 1) x (1, 0, 0) in component "L2_RemovableGrate"
sketch "草图3 (6)" plane through (0, 0, 26) normal (0, 0, 1) x (1, 0, 0) in component "L2_RemovableGrate"
  line L0 (259, 60.3) -> (263, 60.3)
  line L1 (263, 60.3) -> (263, 129.7)
  line L2 (263, 129.7) -> (259, 129.7)
  line L3 (259, 129.7) -> (259, 60.3)
  dimension "d529" = 259
  dimension "d531" = 4
  dimension "d532" = 69.4
  constraint horizontal L0
  constraint vertical L1
  constraint horizontal L2
  constraint vertical L3
  measures "d529" horizontal distance of origin L0.start
  measures "d531" horizontal distance of L0.start L0.end
  measures "d532" vertical distance of L0.end L1.end
extrude "Drain slot 2''" cut sketch "草图3 (6)" along normal blind 4 bodies 6 in component "L2_RemovableGrate"
ref_plane "工作平面4" through (0, 0, 26) normal (0, 0, 1) x (1, 0, 0) in component "L2_RemovableGrate"
sketch "草图4 (6)" plane through (0, 0, 26) normal (0, 0, 1) x (1, 0, 0) in component "L2_RemovableGrate"
  line L0 (269, 60.3) -> (273, 60.3)
  line L1 (273, 60.3) -> (273, 129.7)
  line L2 (273, 129.7) -> (269, 129.7)
  line L3 (269, 129.7) -> (269, 60.3)
  dimension "d537" = 269
  dimension "d539" = 4
  dimension "d540" = 69.4
  constraint horizontal L0
  constraint vertical L1
  constraint horizontal L2
  constraint vertical L3
  measures "d537" horizontal distance of origin L0.start
  measures "d539" horizontal distance of L0.start L0.end
  measures "d540" vertical distance of L0.end L1.end
extrude "Drain slot 3''" cut sketch "草图4 (6)" along normal blind 4 bodies 6 in component "L2_RemovableGrate"
ref_plane "工作平面5" through (0, 0, 26) normal (0, 0, 1) x (1, 0, 0) in component "L2_RemovableGrate"
sketch "草图5 (6)" plane through (0, 0, 26) normal (0, 0, 1) x (1, 0, 0) in component "L2_RemovableGrate"
  line L0 (279, 60.3) -> (283, 60.3)
  line L1 (283, 60.3) -> (283, 129.7)
  line L2 (283, 129.7) -> (279, 129.7)
  line L3 (279, 129.7) -> (279, 60.3)
  dimension "d545" = 279
  dimension "d547" = 4
  dimension "d548" = 69.4
  constraint horizontal L0
  constraint vertical L1
  constraint horizontal L2
  constraint vertical L3
  measures "d545" horizontal distance of origin L0.start
  measures "d547" horizontal distance of L0.start L0.end
  measures "d548" vertical distance of L0.end L1.end
extrude "Drain slot 4''" cut sketch "草图5 (6)" along normal blind 4 bodies 6 in component "L2_RemovableGrate"
ref_plane "工作平面6" through (0, 0, 26) normal (0, 0, 1) x (1, 0, 0) in component "L2_RemovableGrate"
sketch "草图6 (6)" plane through (0, 0, 26) normal (0, 0, 1) x (1, 0, 0) in component "L2_RemovableGrate"
  line L0 (289, 60.3) -> (293, 60.3)
  line L1 (293, 60.3) -> (293, 129.7)
  line L2 (293, 129.7) -> (289, 129.7)
  line L3 (289, 129.7) -> (289, 60.3)
  dimension "d553" = 289
  dimension "d555" = 4
  dimension "d556" = 69.4
  constraint horizontal L0
  constraint vertical L1
  constraint horizontal L2
  constraint vertical L3
  measures "d553" horizontal distance of origin L0.start
  measures "d555" horizontal distance of L0.start L0.end
  measures "d556" vertical distance of L0.end L1.end
extrude "Drain slot 5''" cut sketch "草图6 (6)" along normal blind 4 bodies 6 in component "L2_RemovableGrate"
ref_plane "工作平面7" through (0, 0, 26) normal (0, 0, 1) x (1, 0, 0) in component "L2_RemovableGrate"
sketch "草图7 (6)" plane through (0, 0, 26) normal (0, 0, 1) x (1, 0, 0) in component "L2_RemovableGrate"
  line L0 (299, 60.3) -> (303, 60.3)
  line L1 (303, 60.3) -> (303, 129.7)
  line L2 (303, 129.7) -> (299, 129.7)
  line L3 (299, 129.7) -> (299, 60.3)
  dimension "d561" = 299
  dimension "d563" = 4
  dimension "d564" = 69.4
  constraint horizontal L0
  constraint vertical L1
  constraint horizontal L2
  constraint vertical L3
  measures "d561" horizontal distance of origin L0.start
  measures "d563" horizontal distance of L0.start L0.end
  measures "d564" vertical distance of L0.end L1.end
extrude "Drain slot 6''" cut sketch "草图7 (6)" along normal blind 4 bodies 6 in component "L2_RemovableGrate"
ref_plane "工作平面8" through (0, 0, 26) normal (0, 0, 1) x (1, 0, 0) in component "L2_RemovableGrate"
sketch "草图8 (6)" plane through (0, 0, 26) normal (0, 0, 1) x (1, 0, 0) in component "L2_RemovableGrate"
  line L0 (309, 60.3) -> (313, 60.3)
  line L1 (313, 60.3) -> (313, 129.7)
  line L2 (313, 129.7) -> (309, 129.7)
  line L3 (309, 129.7) -> (309, 60.3)
  dimension "d569" = 309
  dimension "d571" = 4
  dimension "d572" = 69.4
  constraint horizontal L0
  constraint vertical L1
  constraint horizontal L2
  constraint vertical L3
  measures "d569" horizontal distance of origin L0.start
  measures "d571" horizontal distance of L0.start L0.end
  measures "d572" vertical distance of L0.end L1.end
extrude "Drain slot 7''" cut sketch "草图8 (6)" along normal blind 4 bodies 6 in component "L2_RemovableGrate"
ref_plane "工作平面9" through (0, 0, 26) normal (0, 0, 1) x (1, 0, 0) in component "L2_RemovableGrate"
sketch "草图9 (3)" plane through (0, 0, 26) normal (0, 0, 1) x (1, 0, 0) in component "L2_RemovableGrate"
  line L0 (319, 60.3) -> (323, 60.3)
  line L1 (323, 60.3) -> (323, 129.7)
  line L2 (323, 129.7) -> (319, 129.7)
  line L3 (319, 129.7) -> (319, 60.3)
  dimension "d577" = 319
  dimension "d579" = 4
  dimension "d580" = 69.4
  constraint horizontal L0
  constraint vertical L1
  constraint horizontal L2
  constraint vertical L3
  measures "d577" horizontal distance of origin L0.start
  measures "d579" horizontal distance of L0.start L0.end
  measures "d580" vertical distance of L0.end L1.end
extrude "Drain slot 8''" cut sketch "草图9 (3)" along normal blind 4 bodies 6 in component "L2_RemovableGrate"
ref_plane "工作平面10" through (0, 0, 26) normal (0, 0, 1) x (1, 0, 0) in component "L2_RemovableGrate"